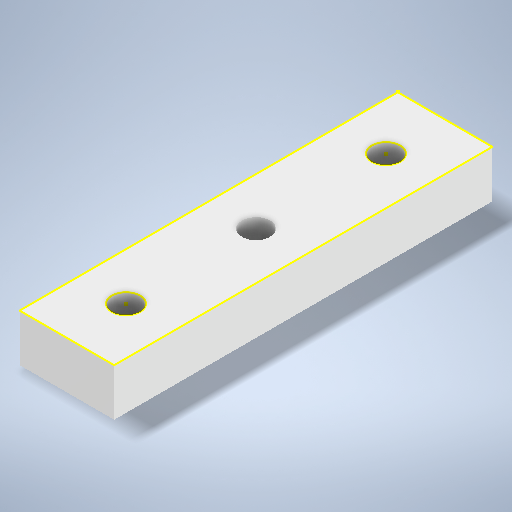
# Autodesk Inventor part: Base mounting to extrusion
Saved by Autodesk Inventor 2025.2 (Build 292293000, 293)
## iProperties
Created: 2025-04-01
Part Number: Base mounting to extrusion
Material: PC/ABS Plastic
Document SubType Name: Modeling
Designer: franc
Density: 1.1 g/cm^3
Appearance: Smooth - White
Author: franc
## iProperties of the stored document Base mounting to extrusion_3DPrint.ipt
Created: 2025-04-09
Part Number: Base mounting to extrusion_3DPrint
Material: Generic
Document SubType Name: Modeling
Designer: franc
Density: 1 g/cm^3
Appearance: Default
Author: franc
Autodesk Inventor part; units mm, degrees
ref_plane "YZ Plane" through (0, 0, 0) normal (1, 0, 0) x (0, 1, 0)
ref_plane "XZ Plane" through (0, 0, 0) normal (0, 1, 0) x (-1, 0, 0)
ref_plane "XY Plane" through (0, 0, 0) normal (0, 0, 1) x (1, 0, 0)
sketch "Sketch1" plane through (0, 0, 0) normal (0, 1, 0) x (-1, 0, 0)
  line L0 (0, 0) -> (-20, 0)
  line L1 (-20, 0) -> (-20, 80)
  line L2 (-20, 80) -> (0, 80)
  line L3 (0, 80) -> (0, 0)
  dimension "d0" = 20
  dimension "d1" = 80
  constraints: 8 end point, 2 parallel, 1 horizontal, 1 perpendicular
  measures "d0" distance of L1.end L2.end
  measures "d1" distance of L0.end L1.end
extrude "Extrusion1" add sketch "Sketch1" along normal blind 10
sketch "Sketch2" plane through (0, 10, 0) normal (0, 1, 0) x (1, 0, 0)
  circle A0 centre (10, -67.5) radius 3
  circle A1 centre (10, -12.5) radius 3
  line L0 (0, -80) -> (20, -80) projected
  line L1 (20, 0) -> (0, 0) projected
  point P0 (10, -80)
  point P1 (10, 0)
  dimension "d4" = 6
  dimension "d5" = 6
  dimension "d6" = 12.5
  dimension "d7" = 12.5
  constraints: 2 centre point, 2 midpoint
  measures "d4" diameter of A0
  measures "d5" diameter of A1
  measures "d6" distance of A0.centre point (10, -80)
  measures "d7" distance of A1.centre point (10, 0)
extrude "Extrusion2" cut sketch "Sketch2" against normal through all
sketch "Sketch3" plane through (0, 0, 0) normal (0, -1, 0) x (1, 0, 0)
  circle A0 centre (10, 67.5) radius 3 projected
  circle A1 centre (10, 67.5) radius 4.75
  circle A2 centre (10, 12.5) radius 3 projected
  circle A3 centre (10, 12.5) radius 4.75
  point P0 (0, 0)
  dimension "d10" = 9.5
  dimension "d11" = 9.5
  constraints: 2 centre point, 2 coincident
  measures "d10" diameter of A1
  measures "d11" diameter of A3
extrude "Extrusion3" cut sketch "Sketch3" against normal blind 2
sketch "Sketch4" plane through (0, 0, 0) normal (0, -1, 0) x (1, 0, 0)
  line L0 (20, 80) -> (20, 0) projected
  line L1 (0, 80) -> (20, 80) projected
  point P0 (0, 0)
  point P1 (10, 40)
sketch "Sketch6" plane through (0, 10, 0) normal (0, 1, 0) x (1, 0, 0)
  circle A0 centre (10, -12.5) radius 3 projected
  circle A1 centre (10, -67.5) radius 3 projected
  line L0 (0, -80) -> (20, -80) projected
  line L1 (20, -80) -> (20, 0) projected
  line L2 (20, 0) -> (0, 0) projected
  line L3 (0, 0) -> (0, -80) projected
hole "Hole2" at (10, 0, 40) direction (0, 1, 0) diameter 6 depth 22.931
body "Solid1"
